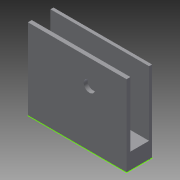
# Autodesk Inventor part: hook diagram
Saved by Autodesk Inventor 2015 (Build 190159000, 159)
## iProperties
Created: 2015-01-12
Part Number: hook diagram
Material: Generic
Document SubType Name: Modeling
Designer: whitaus15
Density: 1 g/cm^3
Appearance: Default
Author: whitaus15
Autodesk Inventor part; units mm, degrees
ref_plane "YZ Plane" through (0, 0, 0) normal (1, 0, 0) x (0, 1, 0)
ref_plane "XZ Plane" through (0, 0, 0) normal (0, 1, 0) x (-1, 0, 0)
ref_plane "XY Plane" through (0, 0, 0) normal (0, 0, 1) x (1, 0, 0)
sketch "Sketch1" plane through (0, 0, 0) normal (0, 1, 0) x (-1, 0, 0)
  line L0 (0, 2.9392) -> (6.6347, 2.9392)
  line L1 (6.6347, 2.9392) -> (6.6347, 0)
  line L2 (6.6347, 0) -> (0, 0)
  line L3 (6.6347, 0) -> (6.6347, -0.4755)
  line L4 (6.6347, -0.4755) -> (0, -0.4755)
  line L5 (6.6347, 2.9392) -> (6.6347, 3.5443)
  line L6 (6.6347, 3.5443) -> (0, 3.5443)
  line L7 (0, 2.9392) -> (-8.8742, 2.9392)
  line L8 (-8.8742, 2.9392) -> (-8.8742, 0)
  line L9 (-8.8742, 0) -> (0, 0)
  line L10 (0, -0.4755) -> (-8.8742, -0.4755)
  line L11 (-8.8742, -0.4755) -> (-8.8742, 0)
  line L12 (0, 3.5443) -> (-8.8742, 3.5443)
  line L13 (-8.8742, 3.5443) -> (-8.8742, 2.9392)
  constraints: 28 end point, 8 perpendicular, 4 point on line, 2 horizontal, 1 collinear, 1 parallel
extrude "Extrusion4" add sketch "Sketch1" along normal blind 12.7 contours L7 L13 L12 L6 L5 L0
extrude "Extrusion5" add sketch "Sketch1" along normal blind 12.7 contours L3 L4 L10 L11 L9 L2
extrude "Extrusion6" add sketch "Sketch1" along normal blind 2.54 contours L0 L1 L2 L9 L8 L7
sketch "Sketch2" plane through (8.8742, 0, -0.4755) normal (0, 0, -1) x (-1, 0, 0)
  circle A0 centre (5.8384, 8.836) radius 0.9005
  point P0 (8.8742, 0)
  constraints: 1 centre point
extrude "Extrusion7" cut sketch "Sketch2" against normal blind 25.4
body "Solid2"
